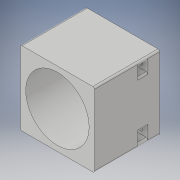
# Autodesk Inventor part: Съёмное крепление мотора 37мм
Saved by Autodesk Inventor 2019.1 (Build 231200000, 200)
## iProperties
Created: 2018-08-01
Part Number: Съёмное крепление мотора 37мм
Material: Типовые
Document SubType Name: Modeling
Designer: olege
Density: 1 g/cm^3
Appearance: По умолчанию
Author: olege
Autodesk Inventor part; units mm, degrees
ref_plane "YZ Plane" through (0, 0, 0) normal (1, 0, 0) x (0, 1, 0)
sketch "Эскиз1" plane through (0, 0, 0) normal (0, 0, 1) x (1, 0, 0)
  line L0 (21.85, -21.85) -> (-21.85, -21.85)
  line L1 (-21.85, -21.85) -> (-21.85, 21.85)
  line L2 (-21.85, 21.85) -> (21.85, 21.85)
  line L3 (21.85, 21.85) -> (21.85, -21.85)
  line L4 (21.85, -21.85) -> (-21.85, 21.85) construction
  line L5 (-21.85, -21.85) -> (21.85, 21.85) construction
  point P0 (0, 0)
  dimension "d0" = 43.7
  dimension "d1" = 43.7
  constraints: 12 end point, 2 midpoint, 2 parallel, 1 horizontal, 1 perpendicular
  measures "d0" distance of L1.end L2.end
  measures "d1" distance of L0.end L1.end
extrude "Выдавливание1" add sketch "Эскиз1" along normal blind 38.5
sketch "Эскиз2" plane through (0, 0, 38.5) normal (0, 0, 1) x (1, 0, 0)
  circle A0 centre (0, 0) radius 18.7
  dimension "d4" = 37.4
  constraints: 1 centre point, 1 coincident
  measures "d4" diameter of A0
extrude "Выдавливание2" cut sketch "Эскиз2" against normal blind 35
sketch "Эскиз3" plane through (0, 0, 3.5) normal (0, 0, 1) x (1, 0, 0)
  circle A0 centre (7, 0) radius 6.2
  circle A1 centre (0, 15.5) radius 1.5
  circle A2 centre (-13.4234, 7.75) radius 1.5
  circle A3 centre (-13.4234, -7.75) radius 1.5
  circle A4 centre (0, -15.5) radius 1.5
  circle A5 centre (13.4234, -7.75) radius 1.5
  circle A6 centre (13.4234, 7.75) radius 1.5
  point P0 (0, 0)
  dimension "d7" = 12.4
  dimension "d8" = 7
  dimension "d9" = 3
  dimension "d10" = 15.5
  dimension "d13" = 360
  constraints: 7 centre point, 1 horizontal alignment, 1 vertical alignment, 13 other
  measures "d7" diameter of A0
  measures "d8" distance of point (0, 0) A0.centre
  measures "d9" diameter of A1
  measures "d10" distance of point (0, 0) A1.centre
extrude "Выдавливание3" cut sketch "Эскиз3" against normal blind 35
chamfer "Фаска1" distance 2 angle 45 6 edges at (-14.9234, -7.75, 0) (-14.9234, 7.75, 0) (-1.5, 15.5, 0) (11.9234, 7.75, 0) (11.9234, -7.75, 0) (-1.5, -15.5, 0)
ref_plane "РабПлоскость1" through (-22.5, 27, -3) normal (0, 1, 0) x (0, 0, 1)
ref_plane "РабПлоскость3" through (0, 0, 7) normal (0, 0, -1) x (-1, 0, 0)
sketch "Эскиз10" plane through (0, 0, 7) normal (0, 0, -1) x (-1, 0, 0)
  line L0 (19.0891, 19.85) -> (20.85, 16.8)
  line L1 (20.85, 16.8) -> (19.0891, 13.75)
  line L2 (19.0891, 13.75) -> (15.5672, 13.75)
  line L3 (15.5672, 13.75) -> (13.8063, 16.8)
  line L4 (13.8063, 16.8) -> (15.5672, 19.85)
  line L5 (15.5672, 19.85) -> (19.0891, 19.85)
  line L6 (21.85, 21.85) -> (-21.85, 21.85) projected
  line L7 (21.85, -21.85) -> (21.85, 21.85) projected
  circle A0 centre (17.3282, 16.8) radius 1.5
  line L8 (-15.5672, 13.75) -> (-19.0891, 13.75)
  line L9 (-19.0891, 13.75) -> (-20.85, 16.8)
  line L10 (-20.85, 16.8) -> (-19.0891, 19.85)
  line L11 (-19.0891, 19.85) -> (-15.5672, 19.85)
  line L12 (-15.5672, 19.85) -> (-13.8063, 16.8)
  line L13 (-13.8063, 16.8) -> (-15.5672, 13.75)
  line L14 (-13.8063, -16.8) -> (-15.5672, -19.85)
  line L15 (-15.5672, -19.85) -> (-19.0891, -19.85)
  line L16 (-19.0891, -19.85) -> (-20.85, -16.8)
  line L17 (-20.85, -16.8) -> (-19.0891, -13.75)
  line L18 (-19.0891, -13.75) -> (-15.5672, -13.75)
  line L19 (-15.5672, -13.75) -> (-13.8063, -16.8)
  line L20 (15.5672, -13.75) -> (19.0891, -13.75)
  line L21 (19.0891, -13.75) -> (20.85, -16.8)
  line L22 (20.85, -16.8) -> (19.0891, -19.85)
  line L23 (19.0891, -19.85) -> (15.5672, -19.85)
  line L24 (15.5672, -19.85) -> (13.8063, -16.8)
  line L25 (13.8063, -16.8) -> (15.5672, -13.75)
  line L26 (-21.85, -21.85) -> (-21.85, 21.85) projected
  line L27 (21.85, -21.85) -> (-21.85, -21.85) projected
  circle A1 centre (-17.3282, 16.8) radius 1.5
  circle A2 centre (-17.3282, -16.8) radius 1.5
  circle A3 centre (17.3282, -16.8) radius 1.5
  line L28 (19.0891, 19.85) -> (24.5205, 19.85)
  line L29 (24.5205, 19.85) -> (24.5205, 13.75)
  line L30 (24.5205, 13.75) -> (19.0891, 13.75)
  line L31 (-19.0891, 19.85) -> (-24.5913, 19.85)
  line L32 (-24.5913, 19.85) -> (-24.5913, 13.75)
  line L33 (-24.5913, 13.75) -> (-19.0891, 13.75)
  line L34 (-19.0891, -13.75) -> (-27.2955, -13.75)
  line L35 (-27.2955, -13.75) -> (-27.2955, -19.85)
  line L36 (-27.2955, -19.85) -> (-19.0891, -19.85)
  line L37 (19.0891, -13.75) -> (24.7592, -13.75)
  line L38 (24.7592, -13.75) -> (24.7592, -19.85)
  line L39 (24.7592, -19.85) -> (19.0891, -19.85)
  point P0 (0, 0)
  point P1 (19.85, 21.85)
  point P2 (21.85, -19.85)
  point P3 (21.85, 19.85)
  point P4 (19.85, -21.85)
  dimension "d58" = 6.1
  dimension "d59" = 2
  dimension "d60" = 1
  dimension "d61" = 3
  dimension "d62" = 6.1
  dimension "d63" = 6.1
  dimension "d64" = 6.1
  dimension "d65" = 2
  dimension "d66" = 1
  dimension "d67" = 2
  dimension "d68" = 1
  dimension "d69" = 1
  dimension "d70" = 2
  dimension "d71" = 3
  dimension "d72" = 3
  dimension "d73" = 3
  constraints: 72 end point, 8 perpendicular, 6 horizontal, 4 centre point, 4 coincident, 4 point on line, 52 other
  measures "d58" distance between parallel lines of L2 L5
  measures "d59" distance between parallel lines of L6 L5
  measures "d60" distance from line of L7 L0.end
  measures "d61" diameter of A0
  measures "d62" distance between parallel lines of L8 L11
  measures "d63" distance between parallel lines of L15 L18
  measures "d64" distance between parallel lines of L23 L20
  measures "d65" distance between parallel lines of L6 L11
  measures "d66" distance from line of L26 L9.end
  measures "d67" distance between parallel lines of L27 L15
  measures "d68" distance from line of L26 L16.end
  measures "d69" distance from line of L7 L21.end
  measures "d70" distance between parallel lines of L27 L23
  measures "d71" diameter of A1
  measures "d72" diameter of A2
  measures "d73" diameter of A3
extrude "Выдавливание9" cut sketch "Эскиз10" against normal blind 6 contours L28 L7 L30 L1 L0 | L0 L1 L2 L3 L4 L5 | L28 L29 L30 L7 | L37 L38 L39 L7 | L7 L39 L22 L21 L37 | L21 L22 L23 L24 L25 L20 | L31 L10 L9 L33 L26 | L26 L33 L32 L31 | L11 L12 L13 L8 L9 L10 | L34 L17 L16 L36 L26 | L26 L36 L35 L34 | L18 L19 L14 L15 L16 L17 | A0 | A1 | A2 | A3
extrude "Выдавливание10" cut sketch "Эскиз10" along normal blind 7 and the other way blind 16 contours A0 | A1 | A2 | A3
fillet "Сопряжение4" radius 1 8 edges at (-21.85, 19.85, 10) (-21.85, 13.75, 10) (-21.85, -13.75, 10) (-21.85, -19.85, 10) (21.85, 19.85, 10) (21.85, 13.75, 10) (21.85, -13.75, 10) (21.85, -19.85, 10)
fillet "Сопряжение5" radius 1 4 edges at (21.85, 21.85, 19.25) (-21.85, 21.85, 19.25) (21.85, -21.85, 19.25) (-21.85, -21.85, 19.25)
equation "\"d62\" = d58"
equation "\"d63\" = d58"
equation "\"d64\" = d58"
equation "\"d65\" = d59"
equation "\"d66\" = d60"
equation "\"d67\" = d59"
equation "\"d68\" = d60"
equation "\"d69\" = d60"
equation "\"d70\" = d59"
